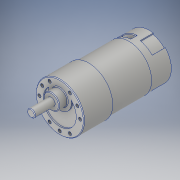
# Autodesk Inventor part: bepf_silnik_dc
Saved by Autodesk Inventor 2017 (Build 210142000, 142)
## iProperties
Created: 2016-11-23
Part Number: bepf_silnik_dc
Material: Aluminium 6061
Document SubType Name: Modeling
Designer: gagato
Density: 2.7 g/cm^3
Appearance: Aluminium — płaski
Mass: 178.515 g
Surface Area: 113.252 cm^2
Volume: 66.1167 cm^3
Author: gagato
Autodesk Inventor part; units mm, degrees
ref_plane "YZ Plane" through (0, 0, 0) normal (1, 0, 0) x (0, 1, 0)
ref_plane "XZ Plane" through (0, 0, 0) normal (0, 1, 0) x (-1, 0, 0)
ref_plane "XY Plane" through (0, 0, 0) normal (0, 0, 1) x (1, 0, 0)
sketch "Szkic1" plane through (0, 0, 0) normal (0, 0, 1) x (1, 0, 0)
  circle A0 centre (0, 0) radius 18.4
  dimension "d0" = 36.8
  constraints: 1 centre point, 1 coincident
  measures "d0" diameter of A0
extrude "Wyciągnięcie proste1" add sketch "Szkic1" against normal blind 22
sketch "Szkic2" plane through (0, 0, -22) normal (0, 0, -1) x (-1, 0, 0)
  circle A0 centre (0, 0) radius 17.4
  dimension "d3" = 34.8
  constraints: 1 centre point, 1 coincident
  measures "d3" diameter of A0
extrude "Wyciągnięcie proste2" add sketch "Szkic2" along normal blind 30.7
sketch "Szkic3" plane through (0, 0, -52.7) normal (0, 0, -1) x (-1, 0, 0)
  circle A0 centre (0, 0) radius 17
  dimension "d6" = 34
  constraints: 1 centre point, 1 coincident
  measures "d6" diameter of A0
extrude "Wyciągnięcie proste3" add sketch "Szkic3" along normal blind 15.4
sketch "Szkic4" plane through (0, 0, 0) normal (0, 0, 1) x (1, 0, 0)
  circle A0 centre (0, 0) radius 12.6
  dimension "d9" = 25.2
  constraints: 1 centre point, 1 coincident
  measures "d9" diameter of A0
extrude "Wyciągnięcie proste4" cut sketch "Szkic4" against normal blind 1
sketch "Szkic5" plane through (0, 0, 0) normal (0, 0, 1) x (1, 0, 0)
  line L0 (0, 0) -> (0, 15.5) construction
  dimension "d12" = 15.5
  constraints: 2 end point, 1 vertical
  measures "d12" distance of L0.start L0.end
hole "Otwór1" at (0, 15.5, 0) direction (0, 0, -1) diameter 2.459 depth 8.8 tip angle 118 thread size "M3x0.5" class "6H" standard "ANSI Metric M Profile"
pattern_circular "Szyk kołowy1" count 3 over 360 about axis through (0, 0, 0) along (0, 0, -1) of "Otwór1"
sketch "Szkic6" plane through (0, 0, 0) normal (0, 0, 1) x (1, 0, 0)
  line L0 (0, 0) -> (-15.5, 0) construction
  dimension "d23" = 15.5
  constraints: 2 end point, 1 horizontal
  measures "d23" distance of L0.start L0.end
hole "Otwór2" at (-15.5, 0, 0) direction (0, 0, -1) diameter 2.459 depth 8.8 tip angle 118 thread size "M3x0.5" class "6H" standard "ANSI Metric M Profile"
pattern_circular "Szyk kołowy2" count 6 over 360 about axis through (0, 0, 0) along (0, 0, -1) of "Otwór2"
sketch "Szkic7" plane through (0, 0, -1) normal (0, 0, 1) x (1, 0, 0)
  line L0 (0, 0) -> (0, -7) construction
  circle A0 centre (0, -7) radius 8.8364
  circle A1 centre (-7.75, -13.4234) radius 1.2295 construction
  dimension "d34" = 7
  constraints: 2 end point, 1 centre point, 1 coincident, 1 tangent, 1 vertical
  measures "d34" distance of L0.start L0.end
extrude "Wyciągnięcie proste5" add sketch "Szkic7" along normal blind 1
sketch "Szkic8" plane through (0, 0, 0) normal (0, 0, 1) x (1, 0, 0)
  line L0 (0, 0) -> (0, -7)
  circle A0 centre (0, -7) radius 6
  dimension "d37" = 7
  dimension "d38" = 12
  constraints: 2 end point, 1 centre point, 1 coincident, 1 vertical
  measures "d37" distance of L0.start L0.end
  measures "d38" diameter of A0
extrude "Wyciągnięcie proste6" add sketch "Szkic8" along normal blind 6.5
sketch "Szkic9" plane through (0, -7, 6.5) normal (0, 0, 1) x (1, 0, 0)
  circle A0 centre (0, 0) radius 6 projected
  circle A1 centre (0, 0) radius 3
  point P0 (0, 7)
  dimension "d41" = 6
  constraints: 1 centre point, 1 coincident
  measures "d41" diameter of A1
extrude "Wyciągnięcie proste7" add sketch "Szkic9" along normal blind 15.5 contours A1
sketch "Szkic10" plane through (0, 0, 0) normal (1, 0, 0) x (0, 1, 0)
  line L0 (-10, 6.5) -> (-10, 22) projected
  line L1 (-4, 22) -> (-10, 22) projected
  line L2 (-4, 22) -> (-4.6, 22)
  line L3 (-4.6, 22) -> (-4.6, 9.5)
  line L4 (-4.6, 9.5) -> (-4, 9.5)
  line L5 (-4, 9.5) -> (-4, 22)
  point P0 (0, 0)
  dimension "d44" = 0.6
  dimension "d45" = 12.5
  constraints: 8 end point, 2 parallel, 1 horizontal, 1 perpendicular
  measures "d44" distance of L4.end L3.end
  measures "d45" distance of L3.end L2.end
extrude "Wyciągnięcie proste8" cut sketch "Szkic10" along normal mid plane 4.25
sketch "Szkic13" plane through (0, 0, -68.1) normal (0, 0, -1) x (-1, 0, 0)
  arc A0 (3, -15.7162) -> (11.6648, -10.9513) centre (0, 0) ccw
  line L0 (0, 0) -> (11.6648, -10.9513) construction
  line L1 (0, 0) -> (3, -15.7162) construction
  arc A1 (3.1875, -16.6985) -> (12.3939, -11.6358) centre (0, 0) ccw
  line L2 (11.6648, -10.9513) -> (12.3939, -11.6358)
  line L3 (3.1875, -16.6985) -> (3, -15.7162)
  dimension "d55" = 16
  dimension "d56" = 36
  dimension "d57" = 3
  dimension "d58" = 17
  dimension "d59" = 36
  constraints: 8 end point, 4 point on circle, 2 centre point, 2 coincident, 1 collinear
  measures "d55" radius of A0
  measures "d56" angle of L1 L0
  measures "d57" horizontal distance of L1.end point (0, 0)
  measures "d58" radius of A1
  measures "d59" angle of L3 L2
extrude "Wyciągnięcie proste10" cut sketch "Szkic13" against normal blind 10
pattern_circular "Szyk kołowy4" count 3 over 360 about axis through (0, 0, -52.7) along (0, 0, -1) of "Wyciągnięcie proste10"
sketch "Szkic14" plane through (0, 0, 0) normal (0, 1, 0) x (-1, 0, 0)
  line L0 (17, -52.7) -> (-17, -52.7) construction
  line L1 (0, -86.12) -> (0, 40.02) construction
  line L2 (-1.5, -59.7) -> (-11.5, -59.7)
  line L3 (-11.5, -59.7) -> (-11.5, -55.7)
  line L4 (-11.5, -55.7) -> (-1.5, -55.7)
  line L5 (-1.5, -55.7) -> (-1.5, -59.7)
  point P0 (0, 0)
  dimension "d65" = 10
  dimension "d66" = 4
  dimension "d67" = 1.5
  dimension "d68" = 3
  constraints: 8 end point, 2 parallel, 1 horizontal, 1 perpendicular
  measures "d65" distance of L3.end L4.end
  measures "d66" distance of L2.end L3.end
  measures "d67" distance between parallel lines of L1 L5
  measures "d68" distance between parallel lines of L0 L4
extrude "Wyciągnięcie proste11" cut sketch "Szkic14" against normal through all
fillet "Zaokrąglenie1" radius 0.5 1 edges at (-6, -7, 6.5)
fillet "Zaokrąglenie2" radius 0.5 2 edges at (-18.4, 0, 0) (-6, -7, 0)
fillet "Zaokrąglenie3" radius 0.5 4 edges at (6.8644, -15.5525, -59.7) (6.8644, -15.5525, -55.7) (11.5, -12.52, -57.7) (1.5, -16.9337, -57.7)
fillet "Zaokrąglenie4" radius 0.5 2 edges at (2.6833, -5.6584, 22) (-1.3416, -9.6833, 22)
move or copy body "Przesuń bryłę1" bodies to move or copy 1 copy no rotation origin (0, 0, 0) rotation axis (0, 0, 1) rotation angle 180
